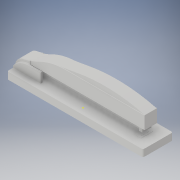
# Autodesk Inventor part: Stapler
Saved by Autodesk Inventor 2017 (Build 210142000, 142)
## iProperties
Created: 2018-03-21
Part Number: Stapler
Material: Generic
Document SubType Name: Modeling
Designer: landontracy
Density: 1 g/cm^3
Appearance: Default
Author: landontracy
Autodesk Inventor part; units mm, degrees
ref_plane "YZ Plane" through (0, 0, 0) normal (1, 0, 0) x (0, 1, 0)
ref_plane "XZ Plane" through (0, 0, 0) normal (0, 1, 0) x (-1, 0, 0)
sketch3d "Stapler Bottom"
  constraints: 16 end point, 2 parallel, 1 horizontal, 1 perpendicular
sketch "Stapler Bottom " plane through (0, 0, 0) normal (0, 1, 0) x (-1, 0, 0)
  line L0 (94.8504, -32.7544) -> (-89.2889, -32.7544)
  line L1 (-90.2889, -31.6958) -> (-90.2889, 7.1831)
  line L2 (-89.8327, 8.1831) -> (94.7084, 8.1831)
  line L3 (95.8504, 7.1831) -> (95.8504, -30.3771)
  line L4 (95.8504, 7.1831) -> (94.7084, 8.1831)
  line L5 (95.8504, -30.3771) -> (94.8504, -32.7544)
  line L6 (-89.2889, -32.7544) -> (-90.2889, -31.6958)
  line L7 (-90.2889, 7.1831) -> (-89.8327, 8.1831)
  point P0 (0, 0)
extrude "Extrusion1" add sketch "Stapler Bottom " along normal blind 9.52
fillet "Fillet1" radius 2 8 edges at (89.8327, 4.76, 8.1831) (90.2889, 4.76, 7.1831) (89.2889, 4.76, -32.7544) (90.2889, 4.76, -31.6958) (-94.8504, 4.76, -32.7544) (-95.8504, 4.76, -30.3771) (-95.8504, 4.76, 7.1831) (-94.7084, 4.76, 8.1831)
sketch "Sketch3" plane through (0, 9.52, 0) normal (0, 1, 0) x (1, 0, 0)
  point P0 (0, 0)
sketch "Sketch4" plane through (0, 9.52, 0) normal (0, 1, 0) x (1, 0, 0)
  line L0 (-95.8504, 29.9736) -> (-95.8504, -6.1831) projected
  line L1 (-95.8504, 0) -> (-73.8768, 0)
  line L2 (-73.8768, 2.5226) -> (-95.8504, 2.5226)
  line L3 (-95.8504, 2.5226) -> (-95.8504, 0)
  line L4 (-95.8504, 11.8953) -> (-84.8636, 11.8953)
  line L5 (-95.8504, 23.7905) -> (-73.8768, 23.7905)
  line L6 (-73.8768, 21.2679) -> (-95.8504, 21.2679)
  line L7 (-95.8504, 21.2679) -> (-95.8504, 23.7905)
  line L8 (-73.8768, 23.7905) -> (-57.9869, 23.7905)
  line L9 (-73.8768, 21.2679) -> (-57.9869, 21.2679)
  line L10 (-57.9869, 21.2679) -> (-57.9869, 23.7905)
  line L11 (-73.8768, 2.5226) -> (-57.9869, 2.5226)
  line L12 (-73.8768, 0) -> (-57.9869, 0)
  line L13 (-57.9869, 0) -> (-57.9869, 2.5226)
  point P0 (0, 0)
  constraints: 26 end point, 6 horizontal, 4 symmetric about line, 3 perpendicular, 1 midpoint, 1 parallel, 1 point on line
extrude "Extrusion2" add sketch "Sketch4" along normal blind 13.175
sketch "Sketch5" plane through (-95.8504, 9.52, 0) normal (0, 0, 1) x (1, 0, 0)
  line L0 (0, 0) -> (0, 13.175) projected
  line L1 (0, 2.7215) -> (7.1075, 13.175)
  line L2 (0, 13.175) -> (37.8635, 13.175) projected
  line L3 (7.1075, 13.175) -> (0, 13.175)
  line L4 (0, 13.175) -> (0, 2.7215)
  point P0 (95.8504, -9.52)
  constraints: 6 end point, 2 point on line, 1 horizontal, 1 perpendicular
extrude "Extrusion3" cut sketch "Sketch5" against normal blind 32.225
fillet "Fillet2" radius 25.8125 2 edges at (-88.7429, 22.695, -1.2613) (-88.7429, 22.695, -22.5292)
sketch "Sketch6" plane through (0, 9.52, 0) normal (0, 1, 0) x (1, 0, 0)
  line L0 (-75.1046, 0) -> (-75.1046, 2.5226) projected
  line L1 (-95.5889, 21.3653) -> (-75.1046, 21.3653)
  line L2 (-75.1046, 21.3653) -> (-75.1046, 2.5226)
  line L3 (-75.1046, 2.5226) -> (-95.5889, 2.5226)
  line L4 (-95.5889, 2.5226) -> (-95.5889, 21.3653)
  point P0 (0, 0)
  constraints: 8 end point, 2 parallel, 1 horizontal, 1 perpendicular
extrude "Extrusion4" add sketch "Sketch6" along normal blind 14.7625
fillet "Fillet3" radius 13.1125 1 edges at (-95.5889, 24.2825, -11.944)
sketch "Sketch7" plane through (-75.1046, 9.52, -2.5226) normal (1, 0, 0) x (0, 0, -1)
  line L0 (0.7655, 13.9146) -> (18.1457, 13.9146)
  line L1 (18.1457, 13.9146) -> (18.1457, 5.7203)
  line L2 (0.7655, 5.7203) -> (0.7655, 13.9146)
  line L3 (0.7655, 10.1654) -> (18.1457, 10.1654)
  point P0 (-2.5226, -9.52)
  constraints: 8 end point, 2 perpendicular, 2 point on line, 1 horizontal, 1 parallel
extrude "Extrusion5" add sketch "Sketch7" along normal blind 156.05
sketch "Sketch8" plane through (-75.1046, 23.4346, -3.2882) normal (0, 1, 0) x (1, 0, 0)
  line L0 (0, 17.3802) -> (156.05, 17.3802) projected
  line L1 (0, 0) -> (156.05, 0) projected
  line L2 (156.05, 17.3802) -> (0, 17.3802)
  line L3 (0, 17.3802) -> (0, 0)
  line L4 (0, 0) -> (156.05, 0)
  line L5 (156.05, 0) -> (156.05, 17.3802)
  point P0 (75.1046, -3.2882)
  constraints: 8 end point, 2 parallel, 1 horizontal, 1 perpendicular
extrude "Extrusion6" add sketch "Sketch8" along normal blind 16.35
fillet "Fillet4" radius 78.2 1 edges at (-75.1046, 39.7846, -11.9783)
fillet "Fillet5" radius 78.2 1 edges at (-75.1046, 24.2825, -11.9783)
fillet "Fillet6" radius 0.4125 9 edges at (-46.6521, 37.6173, -3.2882) (-69.4229, 28.6912, -3.2882) (26.2882, 39.7846, -3.2882) (80.9454, 39.7846, -11.9783) (-46.6521, 37.6173, -20.6684) (-69.4229, 28.6912, -20.6684) (26.2882, 39.7846, -20.6684) (80.9454, 29.735, -3.2882) (80.9454, 29.735, -20.6684)
fillet "Fillet7" radius 0.4125 7 edges at (-66.5457, 22.695, -21.2679) (-86.72, 19.9339, -23.7905) (-66.5457, 22.695, -23.7905) (-86.72, 19.9339, 0) (-66.5457, 22.695, 0) (-66.5457, 22.695, -2.5226) (-86.4593, 20.0635, -2.5226)
fillet "Fillet8" radius 0.4125 1 edges at (-95.8504, 9.52, -11.8953)
fillet "Fillet9" radius 146.4625 1 edges at (-95.5889, 9.52, -11.8953)
sketch "Sketch9" plane through (80.9454, 9.52, -2.5226) normal (1, 0, 0) x (0, 0, -1)
  line L0 (0.7655, 10.1654) -> (0.7655, 16.6266) projected
  line L1 (18.1457, 10.1654) -> (0.7655, 10.1654) projected
  line L2 (18.1457, 12.5223) -> (18.1457, 10.1654)
  line L3 (18.1457, 10.1654) -> (0.7655, 10.1654)
  line L4 (0.7655, 10.1654) -> (0.7655, 12.5223)
  line L5 (0.7655, 12.5223) -> (18.1457, 12.5223)
  line L6 (18.1457, 16.6266) -> (18.1457, 10.1654) projected
  point P0 (-2.5226, -9.52)
  constraints: 8 end point, 1 parallel, 1 perpendicular, 1 point on line
extrude "Extrusion7" cut sketch "Sketch9" against normal blind 156.05
sketch "Sketch10" plane through (80.9454, 22.0423, -20.2559) normal (0, -1, 0) x (1, 0, 0)
  line L0 (-5.4077, 14.5777) -> (-10.1864, 14.5777)
  line L1 (-10.1864, 2.2698) -> (-5.4077, 2.2698)
  line L2 (-5.4077, 2.2698) -> (-5.4077, 14.5777)
  line L3 (-10.1864, 14.5777) -> (-10.1864, 2.2698)
  point P0 (-80.9454, 20.2559)
  constraints: 8 end point, 1 horizontal, 1 parallel
extrude "Extrusion8" add sketch "Sketch10" along normal blind 6.825
sketch "Sketch11" plane through (75.5377, 22.0423, -5.6781) normal (1, 0, 0) x (0, 0, -1)
  line L0 (-2.39, 0) -> (14.9902, 0) projected
  line L1 (0, -6.825) -> (12.3079, -6.825) projected
  circle A0 centre (3.0482, -3.3444) radius 1.2025
  circle A1 centre (9.4058, -3.4806) radius 1.2025
  point P0 (-5.6781, -22.0423)
  constraints: 2 centre point
extrude "Extrusion9" cut sketch "Sketch11" against normal blind 2.0625
sketch "Sketch12" plane through (70.7589, 22.0423, -17.986) normal (-1, 0, 0) x (0, 0, 1)
  point P0 (17.986, -22.0423)
sketch "Sketch13" plane through (70.7589, 22.0423, -17.986) normal (-1, 0, 0) x (0, 0, 1)
  line L0 (12.3079, 0) -> (0, 0) projected
  line L1 (1.5014, 0) -> (1.5014, -5.8244)
  line L2 (1.5014, -5.8244) -> (10.7105, -5.8244)
  line L3 (10.7105, -5.8244) -> (10.7105, 0)
  line L4 (1.5014, 0) -> (10.7105, 0)
  point P0 (17.986, -22.0423)
  constraints: 8 end point, 2 perpendicular, 2 point on line, 1 vertical
extrude "Extrusion10" add sketch "Sketch13" along normal blind 143.35
ref_plane "Work Plane1" through (0, 0, -11.1125) normal (0, 0, 1) x (1, 0, 0)
sketch "Sketch14" plane through (0, 0, -11.1125) normal (0, 0, 1) x (1, 0, 0)
  line L0 (-28.3691, 39.7846) -> (80.5329, 39.7846) projected
  arc A0 (80.5329, 39.7846) -> (-28.3691, 39.7846) centre (26.0819, -166.4003) ccw
  point P0 (0, 0)
  constraints: 2 point on circle, 1 centre point
extrude "Extrusion11" add sketch "Sketch14" along normal mid plane 14.7625
sketch "Sketch15" plane through (0, 0, -18.4938) normal (0, 0, -1) x (-1, 0, 0)
  arc A0 (28.3691, 39.7846) -> (-80.5329, 39.7846) centre (-26.0819, -166.4003) ccw projected
  line L0 (28.3691, 39.7846) -> (-80.5329, 39.7846) projected
  arc A1 (-80.5329, 39.7846) -> (-80.5329, 39.7846) centre (-26.0819, -166.4003) ccw
  point P0 (0, 0)
  constraints: 4 other
extrude "Extrusion12" add sketch "Sketch15" along normal blind 1.5 contours L0 A0
fillet "Fillet10" radius 408.4 1 edges at (-28.3691, 39.7846, -11.8625)
sketch "Sketch16" plane through (0, 9.52, 0) normal (0, 1, 0) x (1, 0, 0)
  point P0 (0, 0)
sketch "Sketch17" plane through (0, 9.52, 0) normal (0, 1, 0) x (1, 0, 0)
  line L0 (75.8483, 20.1912) -> (75.8483, 3.668)
  line L1 (75.8483, 3.668) -> (66.765, 3.668)
  line L2 (66.765, 3.668) -> (66.765, 20.1912)
  line L3 (66.765, 20.1912) -> (75.8483, 20.1912)
  point P0 (0, 0)
  constraints: 8 end point, 3 perpendicular, 1 vertical
extrude "Extrusion13" add sketch "Sketch17" along normal blind 0.3
sketch "Sketch18" plane through (0, 9.82, 0) normal (0, 1, 0) x (1, 0, 0)
  line L0 (75.8483, 20.1912) -> (75.8483, 3.668) projected
  line L1 (66.765, 3.668) -> (66.765, 20.1912) projected
  line L2 (75.8957, 16.9022) -> (75.8957, 14.041)
  line L3 (78.4124, 14.041) -> (78.4124, 16.9022)
  arc A0 (78.4124, 16.9022) -> (75.8957, 16.9022) centre (77.154, 16.9022) ccw
  arc A1 (75.8957, 14.041) -> (78.4124, 14.041) centre (77.154, 14.041) ccw
  line L4 (75.8957, 6.957) -> (75.8957, 9.8182)
  line L5 (78.4124, 9.8182) -> (78.4124, 6.957)
  arc A2 (75.8957, 6.957) -> (78.4124, 6.957) centre (77.154, 6.957) ccw
  arc A3 (78.4124, 9.8182) -> (75.8957, 9.8182) centre (77.154, 9.8182) ccw
  point P0 (0, 0)
  constraints: 8 end point, 8 point on circle, 4 centre point, 2 tangent, 1 parallel
extrude "Extrusion14" cut sketch "Sketch18" against normal blind 0.2
sketch "Sketch19" plane through (80.9454, 15.2173, -20.2559) normal (0, -1, 0) x (1, 0, 0)
  line L0 (-5.4077, 14.5777) -> (-5.4077, 2.2698) projected
  line L1 (-6.2338, 13.3265) -> (-7.8038, 13.3265)
  line L2 (-7.8038, 13.3265) -> (-7.8038, 9.6339)
  line L3 (-7.8038, 9.6339) -> (-6.2338, 9.6339)
  line L4 (-6.2338, 9.6339) -> (-6.2338, 13.3265)
  line L5 (-6.2338, 3.521) -> (-7.8038, 3.521)
  line L6 (-7.8038, 3.521) -> (-7.8038, 7.2136)
  line L7 (-7.8038, 7.2136) -> (-6.2338, 7.2136)
  line L8 (-6.2338, 7.2136) -> (-6.2338, 3.521)
  point P0 (-80.9454, 20.2559)
  constraints: 16 end point, 2 parallel, 1 horizontal, 1 perpendicular
extrude "Extrusion15" cut sketch "Sketch19" against normal blind 0.2
sketch "Sketch20" plane through (0, 9.82, 0) normal (0, 1, 0) x (1, 0, 0)
  line L0 (75.8483, 20.1912) -> (75.8483, 3.668) projected
  line L1 (66.765, 3.668) -> (66.765, 20.1912) projected
  line L2 (73.1083, 17.3734) -> (73.1083, 14.1568)
  line L3 (74.5195, 14.1568) -> (74.5195, 17.3734)
  arc A0 (74.5195, 17.3734) -> (73.1083, 17.3734) centre (73.8139, 17.3734) ccw
  arc A1 (73.1083, 14.1568) -> (74.5195, 14.1568) centre (73.8139, 14.1568) ccw
  line L4 (73.1083, 6.4859) -> (73.1083, 9.7024)
  line L5 (74.5195, 9.7024) -> (74.5195, 6.4859)
  arc A2 (73.1083, 6.4859) -> (74.5195, 6.4859) centre (73.8139, 6.4859) ccw
  arc A3 (74.5195, 9.7024) -> (73.1083, 9.7024) centre (73.8139, 9.7024) ccw
  point P0 (0, 0)
  constraints: 8 end point, 8 point on circle, 4 centre point, 2 tangent, 1 parallel
extrude "Extrusion16" cut sketch "Sketch20" against normal blind 0.2
body "Solid1"
